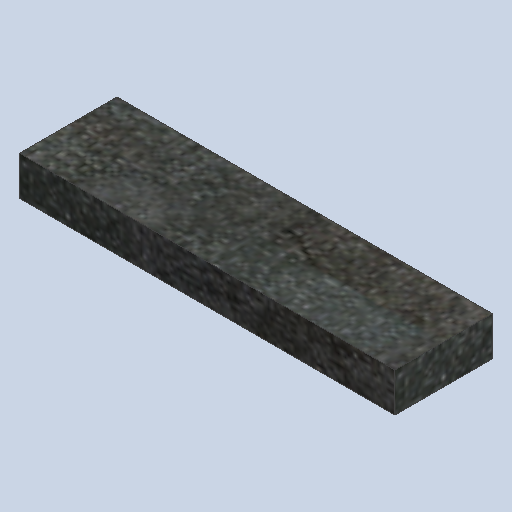
# Autodesk Inventor part: Spannbacke
Saved by Autodesk Inventor 2023.2 (Build 272271000, 271)
## iProperties
Created: 2023-02-07
Part Number: Spannbacke
Material: Steel
Document SubType Name: Modeling
Designer: Ayush
Density: 7.85 g/cm^3
Appearance: Plate
Author: Ayush
Autodesk Inventor part; units mm, degrees
ref_plane "YZ Plane" through (0, 0, 0) normal (1, 0, 0) x (0, 1, 0)
ref_plane "XZ Plane" through (0, 0, 0) normal (0, 1, 0) x (-1, 0, 0)
ref_plane "XY Plane" through (0, 0, 0) normal (0, 0, 1) x (1, 0, 0)
sketch "Sketch1" plane through (0, 0, 0) normal (0, 1, 0) x (-1, 0, 0)
  line L0 (-38.5, 10) -> (38.5, 10)
  line L1 (38.5, 10) -> (38.5, -10)
  line L2 (38.5, -10) -> (-38.5, -10)
  line L3 (-38.5, -10) -> (-38.5, 10)
  line L4 (-38.5, 10) -> (38.5, -10) construction
  line L5 (38.5, 10) -> (-38.5, -10) construction
  circle A0 centre (27.5066, 0) radius 2.5
  circle A1 centre (-27.4934, 0) radius 2.5
  point P0 (0, 0)
  dimension "d0" = 77
  dimension "d1" = 20
  dimension "d2" = 5
  dimension "d3" = 5
  dimension "d4" = 55
  dimension "d5" = 10
  constraints: 12 end point, 2 centre point, 2 midpoint, 2 parallel, 1 horizontal, 1 horizontal alignment, 1 perpendicular
  measures "d0" distance of L1.end L2.end
  measures "d1" distance of L0.end L1.end
  measures "d2" diameter of A0
  measures "d3" diameter of A1
  measures "d4" distance of A1.centre A0.centre
  measures "d5" distance from line of A0.centre L0
extrude "Extrusion1" add sketch "Sketch1" along normal blind 6
sketch "Sketch2" plane through (0, 6, 0) normal (0, 1, 0) x (1, 0, 0)
  line L0 (38.5, 10) -> (-38.5, 10) projected
  line L1 (38.5, -10) -> (-38.5, -10)
  line L2 (-38.5, -10) -> (-38.5, 10)
  line L3 (-38.5, 10) -> (38.5, 10)
  line L4 (38.5, 10) -> (38.5, -10)
  line L5 (38.5, -10) -> (-38.5, 10) construction
  line L6 (-38.5, -10) -> (38.5, 10) construction
  point P0 (0, 0)
  constraints: 12 end point, 2 midpoint, 2 parallel, 1 horizontal, 1 perpendicular
extrude "Extrusion2" add sketch "Sketch2" along normal blind 2
body "Solid1"
